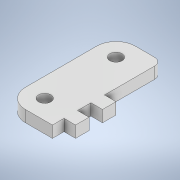
# Autodesk Inventor part: camMountBracket
Saved by Autodesk Inventor 2020 (Build 240168000, 168)
## iProperties
Created: 2019-08-05
Part Number: camMountBracket
Material: Generic
Document SubType Name: Modeling
Designer: n10208577
Density: 1 g/cm^3
Appearance: Default
Author: n10208577
Autodesk Inventor part; units mm, degrees
ref_plane "YZ Plane" through (0, 0, 0) normal (1, 0, 0) x (0, 1, 0)
ref_plane "XZ Plane" through (0, 0, 0) normal (0, 1, 0) x (-1, 0, 0)
ref_plane "XY Plane" through (0, 0, 0) normal (0, 0, 1) x (1, 0, 0)
sketch "Sketch1" plane through (0, 0, 0) normal (0, 1, 0) x (-1, 0, 0)
  circle A0 centre (4.7704, 13.5183) radius 1.6
  circle A1 centre (4.7704, -4.9817) radius 1.6
  line L0 (-5.2296, 5.0183) -> (-2.2296, 5.0183)
  line L1 (-5.2296, 15.5183) -> (-2.2296, 15.5183)
  line L2 (-5.2296, 8.5183) -> (-2.2296, 8.5183)
  line L3 (-5.2296, 12.0183) -> (-2.2296, 12.0183)
  line L4 (-5.2296, 5.0183) -> (-5.2296, 8.5183)
  line L5 (-5.2296, 12.0183) -> (-5.2296, 15.5183)
  line L6 (-2.2296, 15.5183) -> (-2.2296, 18.5183)
  line L7 (-2.2296, 5.0183) -> (-2.2296, -7.9817)
  line L8 (-2.2296, 8.5183) -> (-2.2296, 12.0183)
  line L9 (-2.2296, 18.5183) -> (4.7704, 18.5183)
  arc A2 (9.7704, 13.5183) -> (4.7704, 18.5183) centre (4.7704, 13.5183) ccw
  line L10 (9.7704, 13.5183) -> (9.7704, -4.9817)
  arc A3 (4.7704, -9.9817) -> (9.7704, -4.9817) centre (4.7704, -4.9817) ccw
  line L11 (4.7704, -9.9817) -> (-0.2296, -9.9817)
  arc A4 (-2.2296, -7.9817) -> (-0.2296, -9.9817) centre (-0.2296, -7.9817) ccw
  point P0 (0, 0)
  constraints: 24 end point, 6 point on circle, 5 centre point
extrude "Extrusion1" add sketch "Sketch1" along normal blind 3
body "Solid1"
